Otrio 1_v9 (Autodesk Fusion 360 design; units mm, degrees)
Autodesk Fusion 360 part; units mm, degrees
ref_plane "WorkPlane1" through (0, 0, 6.2) normal (0, 0, 1) x (1, 0, 0)
sketch "Main Sketch1" plane through (0, 0, 6.2) normal (0, 0, 1) x (1, 0, 0)
  circle A0 centre (0, 0) radius 4
  circle A1 centre (0, 0) radius 7
  circle A2 centre (0, 0) radius 10.5
  circle A3 centre (0, 0) radius 15.5
  circle A4 centre (0, 0) radius 19
  circle A5 centre (-43, -86) radius 7
  circle A6 centre (-43, -86) radius 19
  circle A7 centre (-43, -86) radius 4
  circle A8 centre (-43, -86) radius 15.5
  circle A9 centre (-43, -86) radius 10.5
  circle A10 centre (0, -86) radius 7
  circle A11 centre (0, -86) radius 19
  circle A12 centre (0, -86) radius 4
  circle A13 centre (0, -86) radius 15.5
  circle A14 centre (0, -86) radius 10.5
  circle A15 centre (43, -86) radius 7
  circle A16 centre (43, -86) radius 19
  circle A17 centre (43, -86) radius 4
  circle A18 centre (43, -86) radius 15.5
  circle A19 centre (43, -86) radius 10.5
  circle A20 centre (-86, -43) radius 7
  circle A21 centre (-86, -43) radius 19
  circle A22 centre (-86, -43) radius 4
  circle A23 centre (-86, -43) radius 15.5
  circle A24 centre (-86, -43) radius 10.5
  circle A25 centre (-43, -43) radius 7
  circle A26 centre (-43, -43) radius 19
  circle A27 centre (-43, -43) radius 4
  circle A28 centre (-43, -43) radius 15.5
  circle A29 centre (-43, -43) radius 10.5
  circle A30 centre (0, -43) radius 7
  circle A31 centre (0, -43) radius 19
  circle A32 centre (0, -43) radius 4
  circle A33 centre (0, -43) radius 15.5
  circle A34 centre (0, -43) radius 10.5
  circle A35 centre (43, -43) radius 7
  circle A36 centre (43, -43) radius 19
  circle A37 centre (43, -43) radius 4
  circle A38 centre (43, -43) radius 15.5
  circle A39 centre (43, -43) radius 10.5
  circle A40 centre (86, -43) radius 7
  circle A41 centre (86, -43) radius 19
  circle A42 centre (86, -43) radius 4
  circle A43 centre (86, -43) radius 15.5
  circle A44 centre (86, -43) radius 10.5
  circle A45 centre (-86, 0) radius 7
  circle A46 centre (-86, 0) radius 19
  circle A47 centre (-86, 0) radius 4
  circle A48 centre (-86, 0) radius 15.5
  circle A49 centre (-86, 0) radius 10.5
  circle A50 centre (-43, 0) radius 7
  circle A51 centre (-43, 0) radius 19
  circle A52 centre (-43, 0) radius 4
  circle A53 centre (-43, 0) radius 15.5
  circle A54 centre (-43, 0) radius 10.5
  circle A55 centre (43, 0) radius 7
  circle A56 centre (43, 0) radius 19
  circle A57 centre (43, 0) radius 4
  circle A58 centre (43, 0) radius 15.5
  circle A59 centre (43, 0) radius 10.5
  circle A60 centre (86, 0) radius 7
  circle A61 centre (86, 0) radius 19
  circle A62 centre (86, 0) radius 4
  circle A63 centre (86, 0) radius 15.5
  circle A64 centre (86, 0) radius 10.5
  circle A65 centre (-86, 43) radius 7
  circle A66 centre (-86, 43) radius 19
  circle A67 centre (-86, 43) radius 4
  circle A68 centre (-86, 43) radius 15.5
  circle A69 centre (-86, 43) radius 10.5
  circle A70 centre (-43, 43) radius 7
  circle A71 centre (-43, 43) radius 19
  circle A72 centre (-43, 43) radius 4
  circle A73 centre (-43, 43) radius 15.5
  circle A74 centre (-43, 43) radius 10.5
  circle A75 centre (0, 43) radius 7
  circle A76 centre (0, 43) radius 19
  circle A77 centre (0, 43) radius 4
  circle A78 centre (0, 43) radius 15.5
  circle A79 centre (0, 43) radius 10.5
  circle A80 centre (43, 43) radius 7
  circle A81 centre (43, 43) radius 19
  circle A82 centre (43, 43) radius 4
  circle A83 centre (43, 43) radius 15.5
  circle A84 centre (43, 43) radius 10.5
  circle A85 centre (86, 43) radius 7
  circle A86 centre (86, 43) radius 19
  circle A87 centre (86, 43) radius 4
  circle A88 centre (86, 43) radius 15.5
  circle A89 centre (86, 43) radius 10.5
  circle A90 centre (-43, 86) radius 7
  circle A91 centre (-43, 86) radius 19
  circle A92 centre (-43, 86) radius 4
  circle A93 centre (-43, 86) radius 15.5
  circle A94 centre (-43, 86) radius 10.5
  circle A95 centre (0, 86) radius 7
  circle A96 centre (0, 86) radius 19
  circle A97 centre (0, 86) radius 4
  circle A98 centre (0, 86) radius 15.5
  circle A99 centre (0, 86) radius 10.5
  circle A100 centre (43, 86) radius 7
  circle A101 centre (43, 86) radius 19
  circle A102 centre (43, 86) radius 4
  circle A103 centre (43, 86) radius 15.5
  circle A104 centre (43, 86) radius 10.5
  line L0 (65, 65) -> (-65, 65)
  line L1 (-65, 65) -> (-65, -65)
  line L2 (-65, -65) -> (65, -65)
  line L3 (65, -65) -> (65, 65)
  dimension "d1" = 8
  dimension "d2" = 14
  dimension "d3" = 21
  dimension "d4" = 31
  dimension "d5" = 38
  dimension "d8" = 43
  dimension "d9" = 43
  dimension "d50" = 130
  dimension "d51" = 130
  constraint concentric A0 A1
  constraint concentric A1 A2
  constraint concentric A1 A3
  constraint concentric A3 A4
  constraint horizontal L0
  constraint perpendicular L0 L1
  constraint parallel L0 L2
  constraint parallel L1 L3
  constraint coincident A0.centre A1.centre
  measures "d1" diameter of A0
  measures "d2" diameter of A1
  measures "d3" diameter of A2
  measures "d4" diameter of A3
  measures "d5" diameter of A4
  measures "d50" distance of L1 L3
  measures "d51" distance of L0 L2
ref_plane "WorkPlane2" through (0, 0, 8.7) normal (0, 0, 1) x (1, 0, 0)
sketch "dan text" plane through (0, 0, 8.7) normal (0, 0, 1) x (1, 0, 0)
  line L0 (-96.476, -77.9691) -> (-77.8352, -100.1844) construction
  line L1 (-77.8352, -100.1844) -> (-65.5785, -89.8998) construction
  line L2 (-65.5785, -89.8998) -> (-84.2193, -67.6845) construction
  line L3 (-84.2193, -67.6845) -> (-96.476, -77.9691) construction
  dimension "d53" = 7
sketch "base" plane through (0, 0, 0) normal (0, 0, 1) x (1, 0, 0)
  line L0 (69, 111.5) -> (-69, 111.5)
  line L1 (-111.5, 69) -> (-111.5, -69)
  line L2 (-69, -111.5) -> (69, -111.5)
  line L3 (111.5, 111.5) -> (-111.5, -111.5) construction
  line L4 (-111.5, 111.5) -> (111.5, -111.5) construction
  arc A0 (-111.5, 69) -> (-69, 111.5) centre (-111.5, 111.5) ccw
  arc A1 (69, 111.5) -> (111.5, 69) centre (111.5, 111.5) ccw
  arc A2 (111.5, -69) -> (69, -111.5) centre (111.5, -111.5) ccw
  arc A3 (-69, -111.5) -> (-111.5, -69) centre (-111.5, -111.5) ccw
  line L5 (111.5, 69) -> (111.5, -69)
  dimension "d44" = 223
  dimension "d45" = 223
  dimension "d46" = 85
  dimension "d47" = 85
  dimension "d48" = 85
  dimension "d49" = 85
  constraint horizontal L0
  constraint perpendicular L0 L1
  constraint parallel L0 L2
  constraint coincident L3 origin
  constraint coincident L4 origin
  constraint coincident L3.end A3.centre
  constraint coincident L4.end A2.centre
  constraint coincident L3.start A1.centre
  constraint coincident L4.start A0.centre
  measures "d44" distance of L3.end L4.end
  measures "d45" distance of L4.start L3.end
  measures "d46" diameter of A3
  measures "d47" diameter of A2
  measures "d48" diameter of A1
  measures "d49" diameter of A0
extrude "extrude main body" add sketch "base" along normal blind 9.7
extrude "cut groves" cut sketch "Main Sketch1" along normal blind 3.5 contours A0 | A2 | A4 | A6 | A7 | A9 | A11 | A12 | A14 | A16 | A17 | A19 | A21 | A22 | A24 | A26 | A27 | A29 | A31 | A32 | A34 | A36 | A37 | A39 | A41 | A42 | A44 | A46 | A47 | A49 | A51 | A52 | A54 | A56 | A57 | A59 | A61 | A62 | A64 | A66 | A67 | A69 | A71 | A72 | A74 | A76 | A77 | A79 | A81 | A82 | A84 | A86 | A87 | A89 | A91 | A92 | A94 | A96 | A97 | A99 | A101 | A102 | A104
equation "height = 9.7 mm"
equation "grooveheight = 3.5 mm"
equation "d27 = height - grooveheight"
equation "d34 = height"
equation "d36 = grooveheight"
equation "d52 = height - 1 mm"
named bodies: "main"
